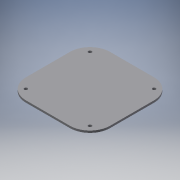
# Autodesk Inventor part: NewFront_D
Saved by Autodesk Inventor 2017 (Build 210142000, 142)
## iProperties
Created: 2019-12-01
Part Number: NewFront_D
Material: Generic
Document SubType Name: Modeling
Designer: DDeGo
Density: 1 g/cm^3
Appearance: Default
Author: DDeGo
Autodesk Inventor part; units mm, degrees
ref_plane "YZ Plane" through (0, 0, 0) normal (1, 0, 0) x (0, 1, 0)
ref_plane "XZ Plane" through (0, 0, 0) normal (0, 1, 0) x (-1, 0, 0)
ref_plane "XY Plane" through (0, 0, 0) normal (0, 0, 1) x (1, 0, 0)
sketch "Sketch1" plane through (0, 0, 0) normal (0, 0, 1) x (1, 0, 0)
  line L0 (-27.45, -52.45) -> (27.45, -52.45)
  line L1 (52.45, -27.45) -> (52.45, 27.45)
  line L2 (27.45, 52.45) -> (-27.45, 52.45)
  line L3 (-52.45, 27.45) -> (-52.45, -27.45)
  line L4 (-52.45, -52.45) -> (52.45, 52.45) construction
  line L5 (52.45, -52.45) -> (-52.45, 52.45) construction
  arc A0 (-27.45, 52.45) -> (-52.45, 27.45) centre (-27.45, 27.45) ccw
  arc A1 (-52.45, -27.45) -> (-27.45, -52.45) centre (-27.45, -27.45) ccw
  arc A2 (27.45, -52.45) -> (52.45, -27.45) centre (27.45, -27.45) ccw
  arc A3 (52.45, 27.45) -> (27.45, 52.45) centre (27.45, 27.45) ccw
  line L6 (-37.5, 37.5) -> (37.5, 37.5) construction
  line L7 (37.5, 37.5) -> (37.5, -37.5) construction
  line L8 (37.5, -37.5) -> (-37.5, -37.5) construction
  line L9 (-37.5, -37.5) -> (-37.5, 37.5) construction
  line L10 (-37.5, 37.5) -> (37.5, -37.5) construction
  line L11 (37.5, 37.5) -> (-37.5, -37.5) construction
  circle A4 centre (37.5, 37.5) radius 2
  circle A5 centre (37.5, -37.5) radius 2
  circle A6 centre (-37.5, -37.5) radius 2
  circle A7 centre (-37.5, 37.5) radius 2
  point P0 (0, 0)
  dimension "d0" = 104.9
  dimension "d1" = 104.9
  dimension "d2" = 25
  dimension "d6" = 75
  dimension "d7" = 4
  constraints: 24 end point, 8 centre point, 8 point on circle, 8 point on line, 8 tangent, 6 equal radius, 4 coincident, 4 midpoint, 4 parallel, 3 perpendicular, 2 horizontal
  measures "d0" distance between parallel lines of L3 L1
  measures "d1" distance between parallel lines of L2 L0
  measures "d2" radius of A0
  measures "d6" distance of L8.end L6.start
  measures "d7" diameter of A4
extrude "Extrusion1" add sketch "Sketch1" along normal blind 2.5
equation "\"d1\" = d0"
body "Solid1"
